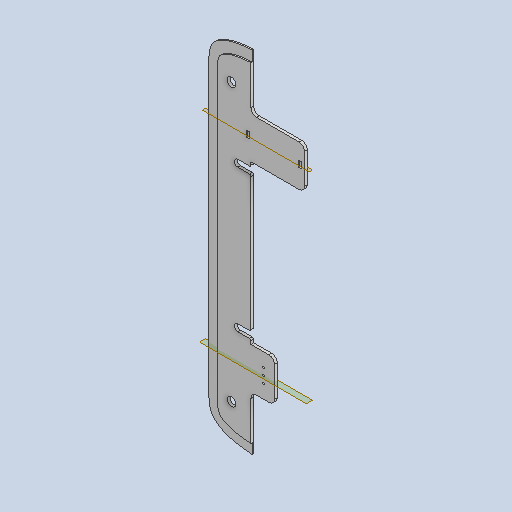
# Autodesk Inventor part: back_led_board
Saved by Autodesk Inventor 2022 (Build 260153000, 153)
## iProperties
Created: 2024-12-22
Part Number: back_led_board
Material: Типовые
Document SubType Name: Modeling
Designer: Andrey
Density: 1 g/cm^3
Appearance: По умолчанию
Author: Andrey
Autodesk Inventor part; units mm, degrees
ref_plane "YZ Plane" through (0, 0, 0) normal (1, 0, 0) x (0, 1, 0)
ref_plane "XZ Plane" through (0, 0, 0) normal (0, 1, 0) x (-1, 0, 0)
ref_plane "XY Plane" through (0, 0, 0) normal (0, 0, 1) x (1, 0, 0)
sketch "Эскиз1" plane through (0, 0, 0) normal (0, 0, 1) x (1, 0, 0)
  arc A0 (21.9698, 25.0872) -> (24.9698, 22.0872) centre (24.9698, 25.0872) ccw
  line L0 (24.9698, 22.0872) -> (32.4715, 22.0872)
  arc A1 (35.4715, 19.0872) -> (32.4715, 22.0872) centre (32.4715, 19.0872) ccw
  line L1 (35.4715, 19.0872) -> (35.4715, -12.1128)
  arc A2 (32.4715, -15.1128) -> (35.4715, -12.1128) centre (32.4715, -12.1128) ccw
  line L2 (32.4715, -15.1128) -> (24.9698, -15.1128)
  arc A3 (24.9698, -15.1128) -> (21.9698, -18.1128) centre (24.9698, -18.1128) ccw
  line L3 (21.9698, -18.1128) -> (21.9698, -28.1128)
  line L4 (21.9698, -28.1128) -> (36.9698, -28.1128)
  line L5 (36.9698, -28.1128) -> (36.9698, -40.6128)
  line L6 (36.9698, -40.6128) -> (21.9698, -40.6128)
  line L7 (21.9698, -40.6128) -> (21.9698, -43.5128)
  line L8 (21.9698, -43.5128) -> (58.0248, -43.5128)
  arc A4 (60.0248, -45.5128) -> (58.0248, -43.5128) centre (58.0248, -45.5128) ccw
  line L9 (60.0248, -45.5128) -> (60.0248, -60.8075)
  arc A5 (58.0248, -62.8075) -> (60.0248, -60.8075) centre (58.0248, -60.8075) ccw
  line L10 (58.0248, -62.8075) -> (-57.9752, -62.8075)
  arc A6 (-59.9752, -60.8075) -> (-57.9752, -62.8075) centre (-57.9752, -60.8075) ccw
  line L11 (-59.9752, -60.8075) -> (-59.9752, -45.5128)
  arc A7 (-57.9752, -43.5128) -> (-59.9752, -45.5128) centre (-57.9752, -45.5128) ccw
  line L12 (-57.9752, -43.5128) -> (-22.0457, -43.5128)
  line L13 (-22.0457, -43.5128) -> (-22.0457, -40.6128)
  line L14 (-22.0457, -40.6128) -> (-39.5957, -40.6128)
  line L15 (-39.5957, -40.6128) -> (-39.5957, -29.6128)
  line L16 (-39.5957, -29.6128) -> (-22.0457, -29.6128)
  line L17 (-22.0457, -29.6128) -> (-22.0457, -27.6266)
  line L18 (-22.0457, -27.6266) -> (-23.1715, -27.6266)
  line L19 (-23.1715, -27.6266) -> (-23.1715, -10.2508)
  line L20 (-23.1715, -10.2508) -> (-22.0457, -10.2508)
  line L21 (-22.0457, -10.2508) -> (-22.0457, -5.0128)
  line L22 (-22.0457, -5.0128) -> (-25.0457, -5.0128)
  line L23 (-25.0457, -5.0128) -> (-25.0457, 4.9872)
  line L24 (-25.0457, 4.9872) -> (-22.0457, 4.9872)
  line L25 (-22.0457, 4.9872) -> (-22.0457, 10.2252)
  line L26 (-22.0457, 10.2252) -> (-23.1715, 10.2252)
  line L27 (-23.1715, 10.2252) -> (-23.1715, 27.601)
  line L28 (-23.1715, 27.601) -> (-22.0457, 27.601)
  line L29 (-22.0457, 27.601) -> (-22.0457, 43.4872)
  line L30 (-22.0457, 43.4872) -> (-57.9752, 43.4872)
  arc A8 (-59.9752, 45.4872) -> (-57.9752, 43.4872) centre (-57.9752, 45.4872) ccw
  line L31 (-59.9752, 45.4872) -> (-59.9752, 60.782)
  arc A9 (-57.9752, 62.782) -> (-59.9752, 60.782) centre (-57.9752, 60.782) ccw
  line L32 (-57.9752, 62.782) -> (58.0248, 62.782)
  arc A10 (60.0248, 60.782) -> (58.0248, 62.782) centre (58.0248, 60.782) ccw
  line L33 (60.0248, 60.782) -> (60.0248, 45.4872)
  arc A11 (58.0248, 43.4872) -> (60.0248, 45.4872) centre (58.0248, 45.4872) ccw
  line L34 (58.0248, 43.4872) -> (21.9698, 43.4872)
  line L35 (21.9698, 43.4872) -> (21.9698, 25.0872)
  circle A12 centre (-51.6466, 22.9919) radius 1.5
  circle A13 centre (-51.6466, -23.0174) radius 1.5
  line L36 (-50.445, -3.8128) -> (-50.445, 15.6872)
  arc A14 (-47.445, 18.6872) -> (-50.445, 15.6872) centre (-47.445, 15.6872) ccw
  line L37 (-47.445, 18.6872) -> (-33.6813, 18.6872)
  arc A15 (-30.6813, 15.6872) -> (-33.6813, 18.6872) centre (-33.6813, 15.6872) ccw
  line L38 (-30.6813, 15.6872) -> (-30.6813, -3.8128)
  arc A16 (-33.6813, -6.8128) -> (-30.6813, -3.8128) centre (-33.6813, -3.8128) ccw
  line L39 (-33.6813, -6.8128) -> (-47.445, -6.8128)
  arc A17 (-50.445, -3.8128) -> (-47.445, -6.8128) centre (-47.445, -3.8128) ccw
  line L40 (60.4248, -29.3128) -> (60.4248, -21.9128)
  line L41 (60.4248, -21.9128) -> (74.9248, -21.9128)
  line L42 (74.9248, -21.9128) -> (74.9248, -29.3128)
  line L43 (74.9248, -29.3128) -> (60.4248, -29.3128)
  line L44 (60.4248, 21.8872) -> (60.4248, 29.2872)
  line L45 (60.4248, 29.2872) -> (74.9248, 29.2872)
  line L46 (74.9248, 29.2872) -> (74.9248, 21.8872)
  line L47 (74.9248, 21.8872) -> (60.4248, 21.8872)
  line L48 (79.0248, -17.5128) -> (68.0248, -17.5128)
  line L49 (68.0248, -17.5128) -> (68.0248, -6.0128)
  line L50 (68.0248, -6.0128) -> (63.1715, -6.0128)
  arc A18 (62.1715, -5.0128) -> (63.1715, -6.0128) centre (63.1715, -5.0128) ccw
  line L51 (62.1715, -5.0128) -> (62.1715, 4.9872)
  arc A19 (63.1715, 5.9872) -> (62.1715, 4.9872) centre (63.1715, 4.9872) ccw
  line L52 (63.1715, 5.9872) -> (68.0248, 5.9872)
  line L53 (68.0248, 5.9872) -> (68.0248, 17.4872)
  line L54 (68.0248, 17.4872) -> (79.0248, 17.4872)
  line L55 (79.0248, 17.4872) -> (79.0248, 52.7508)
  spline S0 degree 4 poles (79.0248, 52.7508) (79.0248, 55.4389) (78.6593, 58.1507) (77.2994, 60.4709) (75.0248, 62.2967) knots 0 0 0 0 0 1 1 1 1 1
  spline S1 degree 4 poles (75.0248, 62.2967) (71.8239, 64.8662) (66.8118, 66.4567) (60.2111, 66.782) (55.0248, 66.782) knots 0.415412 0.415412 0.415412 0.415412 0.415412 1 1 1 1 1
  line L56 (-54.9752, 66.782) -> (55.0248, 66.782)
  spline S2 degree 4 poles (-54.9752, 66.782) (-60.1615, 66.782) (-66.7622, 66.4567) (-71.7743, 64.8662) (-74.9752, 62.2967) knots 0 0 0 0 0 0.584588 0.584588 0.584588 0.584588 0.584588
  spline S3 degree 4 poles (-74.9752, 62.2967) (-77.2498, 60.4709) (-78.6098, 58.1507) (-78.9752, 55.4389) (-78.9752, 52.7508) knots 0 0 0 0 0 1 1 1 1 1
  line L57 (-78.9752, 52.7508) -> (-78.9752, -52.7764)
  spline S4 degree 4 poles (-78.9752, -52.7764) (-78.9752, -55.4644) (-78.6098, -58.1763) (-77.2498, -60.4964) (-74.9752, -62.3223) knots 0 0 0 0 0 1 1 1 1 1
  spline S5 degree 4 poles (-74.9752, -62.3223) (-71.7743, -64.8917) (-66.7622, -66.4822) (-60.1615, -66.8075) (-54.9752, -66.8075) knots 0.415412 0.415412 0.415412 0.415412 0.415412 1 1 1 1 1
  line L58 (55.0248, -66.8075) -> (-54.9752, -66.8075)
  spline S6 degree 4 poles (55.0248, -66.8075) (60.2111, -66.8075) (66.8118, -66.4822) (71.8239, -64.8917) (75.0248, -62.3223) knots 0 0 0 0 0 0.584588 0.584588 0.584588 0.584588 0.584588
  spline S7 degree 4 poles (75.0248, -62.3223) (77.2994, -60.4964) (78.6593, -58.1763) (79.0248, -55.4644) (79.0248, -52.7764) knots 0 0 0 0 0 1 1 1 1 1
  line L59 (79.0248, -52.7764) -> (79.0248, -17.5128)
  circle A20 centre (-29.4752, -25.5128) radius 1.25
  circle A21 centre (29.5248, 25.4872) radius 1.25
  circle A22 centre (29.5248, -25.5128) radius 1.25
  circle A23 centre (-29.4752, 25.4872) radius 1.25
  line L60 (-75.6752, -52.7764) -> (-75.6752, 52.7508)
  line L61 (-54.9752, 63.482) -> (55.0248, 63.482)
  line L62 (75.7248, 52.7508) -> (75.7248, 20.7872)
  line L63 (75.7248, 20.7872) -> (64.7248, 20.7872)
  line L64 (64.7248, 20.7872) -> (64.7248, 8.9969)
  arc A24 (64.7248, 8.9969) -> (58.8715, 4.9872) centre (63.1715, 4.9872) ccw
  line L65 (58.8715, 4.9872) -> (58.8715, -5.0128)
  arc A25 (58.8715, -5.0128) -> (64.7248, -9.0224) centre (63.1715, -5.0128) ccw
  line L66 (64.7248, -9.0224) -> (64.7248, -20.8128)
  line L67 (64.7248, -20.8128) -> (75.7248, -20.8128)
  line L68 (75.7248, -20.8128) -> (75.7248, -52.7764)
  line L69 (55.0248, -63.5075) -> (-54.9752, -63.5075)
  line L70 (-78.9752, 52.7508) -> (-78.9752, -52.7764)
  spline S8 degree 4 poles (-78.9752, -52.7764) (-78.9752, -55.4644) (-78.6098, -58.1763) (-77.2498, -60.4964) (-74.9752, -62.3223) knots 0 0 0 0 0 1 1 1 1 1
  spline S9 degree 4 poles (-74.9752, -62.3223) (-72.4991, -64.31) (-68.939, -65.7118) (-64.3981, -66.3953) (-59.9752, -66.667) knots 0 0 0 0 0 1 1 1 1 1
  line L71 (-59.9752, -66.667) -> (-59.9752, -28.4266)
  line L72 (-59.9752, -28.4266) -> (-75.9752, -28.4266)
  line L73 (-75.9752, -28.4266) -> (-75.9752, 28.401)
  line L74 (-75.9752, 28.401) -> (-59.9752, 28.401)
  line L75 (-59.9752, 28.401) -> (-59.9752, 66.6415)
  spline S10 degree 4 poles (-59.9752, 66.6415) (-64.3981, 66.3697) (-68.939, 65.6863) (-72.4991, 64.2844) (-74.9752, 62.2967) knots 0 0 0 0 0 1 1 1 1 1
  spline S11 degree 4 poles (-74.9752, 62.2967) (-77.2498, 60.4709) (-78.6098, 58.1507) (-78.9752, 55.4389) (-78.9752, 52.7508) knots 0 0 0 0 0 1 1 1 1 1
  line L76 (-78.9752, 52.7508) -> (-78.9752, -52.7764)
  spline S12 degree 4 poles (-74.9752, 62.2967) (-77.2498, 60.4709) (-78.6098, 58.1507) (-78.9752, 55.4389) (-78.9752, 52.7508) knots 0 0 0 0 0 1 1 1 1 1
  spline S13 degree 4 poles (-59.9752, 66.6415) (-64.3981, 66.3697) (-68.939, 65.6863) (-72.4991, 64.2844) (-74.9752, 62.2967) knots 0 0 0 0 0 1 1 1 1 1
  line L77 (-59.9752, 63.6356) -> (-59.9752, 66.6415)
  spline S14 degree 3 poles (-73.0972, 59.9572) (-72.8317, 60.1704) (-72.2504, 60.5866) (-71.3901, 61.0754) (-70.4297, 61.5347) (-69.5826, 61.8759) (-68.4322, 62.2648) (-67.4425, 62.5442) (-66.1307, 62.8516) (-65.027, 63.0635) (-63.595, 63.2862) (-62.4143, 63.4312) (-61.1039, 63.5554) (-60.3883, 63.6089) (-59.9752, 63.6356) knots 0 0 0 0 0.108911 0.217823 0.272278 0.38119 0.435645 0.544557 0.599012 0.707924 0.762379 0.871291 0.925747 1 1 1 1
  spline S15 degree 3 poles (-75.9752, 52.7508) (-75.9752, 53.2802) (-75.9431, 54.1752) (-75.8223, 55.1158) (-75.6926, 55.7827) (-75.5863, 56.208) (-75.4279, 56.7161) (-75.2804, 57.1045) (-75.0687, 57.5698) (-74.8765, 57.9272) (-74.6051, 58.3588) (-74.3614, 58.6932) (-74.0195, 59.1004) (-73.638, 59.4977) (-73.2859, 59.8058) (-73.0972, 59.9572) knots 0 0 0 0 0.166667 0.291667 0.333333 0.416667 0.458333 0.541667 0.583333 0.666667 0.708333 0.791667 0.833333 0.916667 1 1 1 1
  line L78 (-75.9752, -52.7764) -> (-75.9752, 52.7508)
  spline S16 degree 3 poles (-73.0972, -59.9828) (-73.2859, -59.8313) (-73.638, -59.5233) (-74.0195, -59.126) (-74.3614, -58.7188) (-74.6051, -58.3843) (-74.8765, -57.9527) (-75.0687, -57.5953) (-75.2804, -57.1301) (-75.4279, -56.7417) (-75.5863, -56.2336) (-75.6926, -55.8083) (-75.8007, -55.2525) (-75.8676, -54.7887) (-75.9281, -54.186) (-75.9662, -53.5615) (-75.9752, -53.0411) (-75.9752, -52.7764) knots 0 0 0 0 0.083333 0.166667 0.208333 0.291667 0.333333 0.416667 0.458333 0.541667 0.583333 0.666667 0.708333 0.791667 0.833333 0.916667 1 1 1 1
  spline S17 degree 3 poles (-59.9752, -63.6611) (-60.3883, -63.6345) (-61.1039, -63.581) (-62.4143, -63.4568) (-63.595, -63.3118) (-65.027, -63.0891) (-66.1307, -62.8772) (-67.4425, -62.5698) (-68.4322, -62.2903) (-69.5826, -61.9014) (-70.4297, -61.5602) (-71.3901, -61.101) (-72.2504, -60.6122) (-72.8317, -60.196) (-73.0972, -59.9828) knots 0 0 0 0 0.074253 0.128709 0.237621 0.292076 0.400988 0.455443 0.564355 0.61881 0.727722 0.782177 0.891089 1 1 1 1
  line L79 (-59.9752, -66.667) -> (-59.9752, -63.6611)
  spline S18 degree 4 poles (-74.9752, -62.3223) (-72.4991, -64.31) (-68.939, -65.7118) (-64.3981, -66.3953) (-59.9752, -66.667) knots 0 0 0 0 0 1 1 1 1 1
  spline S19 degree 4 poles (-78.9752, -52.7764) (-78.9752, -55.4644) (-78.6098, -58.1763) (-77.2498, -60.4964) (-74.9752, -62.3223) knots 0 0 0 0 0 1 1 1 1 1
  line L80 (-59.9752, -66.667) -> (-59.9752, 66.6415)
  spline S20 degree 5 poles (-54.9752, -63.5075) (-57.0934, -63.5074) (-59.2113, -63.4553) (-61.3274, -63.3195) (-65.0377, -62.9091) (-68.6545, -61.9829) (-70.1733, -61.4591) (-71.6562, -60.755) (-72.9094, -59.7489) knots 0 0 0 0 0 0 0.568819 0.568819 0.568819 1 1 1 1 1 1
  spline S21 degree 5 poles (-72.9094, -59.7489) (-73.483, -59.2877) (-74.0084, -58.7674) (-74.4613, -58.1707) (-75.2019, -56.783) (-75.5464, -55.2458) (-75.6371, -54.4235) (-75.6756, -53.6003) (-75.6752, -52.7764) knots 0 0 0 0 0 0 0.47184 0.47184 0.47184 1 1 1 1 1 1
  spline S22 degree 5 poles (-75.6752, 52.7508) (-75.6756, 53.5748) (-75.6371, 54.398) (-75.5464, 55.2203) (-75.2019, 56.7574) (-74.4613, 58.1451) (-74.0084, 58.7418) (-73.483, 59.2621) (-72.9094, 59.7233) knots 0 0 0 0 0 0 0.52816 0.52816 0.52816 1 1 1 1 1 1
  spline S23 degree 5 poles (-72.9094, 59.7233) (-71.6562, 60.7294) (-70.1733, 61.4336) (-68.6545, 61.9574) (-65.0377, 62.8835) (-61.3274, 63.2939) (-59.2113, 63.4297) (-57.0934, 63.4818) (-54.9752, 63.482) knots 0 0 0 0 0 0 0.431181 0.431181 0.431181 1 1 1 1 1 1
  spline S24 degree 5 poles (55.0248, 63.482) (57.143, 63.4818) (59.2609, 63.4297) (61.377, 63.2939) (65.0873, 62.8835) (68.704, 61.9574) (70.2229, 61.4336) (71.7058, 60.7294) (72.959, 59.7233) knots 0 0 0 0 0 0 0.568819 0.568819 0.568819 1 1 1 1 1 1
  spline S25 degree 5 poles (72.959, 59.7233) (73.5326, 59.2621) (74.0579, 58.7418) (74.5109, 58.1451) (75.2514, 56.7574) (75.596, 55.2203) (75.6867, 54.398) (75.7252, 53.5748) (75.7248, 52.7508) knots 0 0 0 0 0 0 0.47184 0.47184 0.47184 1 1 1 1 1 1
  spline S26 degree 5 poles (75.7248, -52.7764) (75.7252, -53.6003) (75.6867, -54.4235) (75.596, -55.2458) (75.2514, -56.783) (74.5109, -58.1707) (74.0579, -58.7674) (73.5326, -59.2877) (72.959, -59.7489) knots 0 0 0 0 0 0 0.52816 0.52816 0.52816 1 1 1 1 1 1
  spline S27 degree 5 poles (72.959, -59.7489) (71.7058, -60.755) (70.2229, -61.4591) (68.704, -61.9829) (65.0873, -62.9091) (61.377, -63.3195) (59.2609, -63.4553) (57.143, -63.5074) (55.0248, -63.5075) knots 0 0 0 0 0 0 0.431181 0.431181 0.431181 1 1 1 1 1 1
  point P0 (0, 0)
  point P1 (-59.9752, -63.3605)
  point P2 (-59.9752, 63.3349)
  dimension "d0" = 3.3
  constraints: 22 end point, 7 parallel, 4 point on circle, 2 centre point, 1 vertical, 32 other
extrude "Выдавливание1" add sketch "Эскиз1" along normal blind 1 contours L31 L75 L74 L60 S22 S23 | L80 L72 L60 L74 | L71 L11 S20 S21 L60 L72
sketch "Эскиз2" plane through (0, 0, 1) normal (0, 0, 1) x (1, 0, 0)
  line L0 (-44.445, -31.1128) -> (-44.445, -39.1128)
  arc A0 (-45.445, -40.1128) -> (-44.445, -39.1128) centre (-45.445, -39.1128) ccw
  line L1 (-45.445, -40.1128) -> (-48.445, -40.1128)
  arc A1 (-49.445, -39.1128) -> (-48.445, -40.1128) centre (-48.445, -39.1128) ccw
  line L2 (-49.445, -39.1128) -> (-49.445, -31.1128)
  arc A2 (-48.445, -30.1128) -> (-49.445, -31.1128) centre (-48.445, -31.1128) ccw
  line L3 (-48.445, -30.1128) -> (-45.445, -30.1128)
  arc A3 (-44.445, -31.1128) -> (-45.445, -30.1128) centre (-45.445, -31.1128) ccw
  circle A4 centre (-29.4752, 25.4872) radius 1.25
  circle A5 centre (29.5248, -25.5128) radius 1.25
  circle A6 centre (29.5248, 25.4872) radius 1.25
  circle A7 centre (-29.4752, -25.5128) radius 1.25
  line L4 (79.0248, -17.5128) -> (68.0248, -17.5128)
  line L5 (68.0248, -17.5128) -> (68.0248, -6.0128)
  line L6 (68.0248, -6.0128) -> (63.1715, -6.0128)
  arc A8 (62.1715, -5.0128) -> (63.1715, -6.0128) centre (63.1715, -5.0128) ccw
  line L7 (62.1715, -5.0128) -> (62.1715, 4.9872)
  arc A9 (63.1715, 5.9872) -> (62.1715, 4.9872) centre (63.1715, 4.9872) ccw
  line L8 (63.1715, 5.9872) -> (68.0248, 5.9872)
  line L9 (68.0248, 5.9872) -> (68.0248, 17.4872)
  line L10 (68.0248, 17.4872) -> (79.0248, 17.4872)
  line L11 (79.0248, 17.4872) -> (79.0248, 52.7508)
  spline S0 degree 4 poles (79.0248, 52.7508) (79.0248, 55.4389) (78.6593, 58.1507) (77.2994, 60.4709) (75.0248, 62.2967) knots 0 0 0 0 0 1 1 1 1 1
  spline S1 degree 4 poles (75.0248, 62.2967) (71.8239, 64.8662) (66.8118, 66.4567) (60.2111, 66.782) (55.0248, 66.782) knots 0.415412 0.415412 0.415412 0.415412 0.415412 1 1 1 1 1
  line L12 (-54.9752, 66.782) -> (55.0248, 66.782)
  spline S2 degree 4 poles (-54.9752, 66.782) (-60.1615, 66.782) (-66.7622, 66.4567) (-71.7743, 64.8662) (-74.9752, 62.2967) knots 0 0 0 0 0 0.584588 0.584588 0.584588 0.584588 0.584588
  spline S3 degree 4 poles (-74.9752, 62.2967) (-77.2498, 60.4709) (-78.6098, 58.1507) (-78.9752, 55.4389) (-78.9752, 52.7508) knots 0 0 0 0 0 1 1 1 1 1
  line L13 (-78.9752, 52.7508) -> (-78.9752, -52.7764)
  spline S4 degree 4 poles (-78.9752, -52.7764) (-78.9752, -55.4644) (-78.6098, -58.1763) (-77.2498, -60.4964) (-74.9752, -62.3223) knots 0 0 0 0 0 1 1 1 1 1
  spline S5 degree 4 poles (-74.9752, -62.3223) (-71.7743, -64.8917) (-66.7622, -66.4822) (-60.1615, -66.8075) (-54.9752, -66.8075) knots 0.415412 0.415412 0.415412 0.415412 0.415412 1 1 1 1 1
  line L14 (55.0248, -66.8075) -> (-54.9752, -66.8075)
  spline S6 degree 4 poles (55.0248, -66.8075) (60.2111, -66.8075) (66.8118, -66.4822) (71.8239, -64.8917) (75.0248, -62.3223) knots 0 0 0 0 0 0.584588 0.584588 0.584588 0.584588 0.584588
  spline S7 degree 4 poles (75.0248, -62.3223) (77.2994, -60.4964) (78.6593, -58.1763) (79.0248, -55.4644) (79.0248, -52.7764) knots 0 0 0 0 0 1 1 1 1 1
  line L15 (79.0248, -52.7764) -> (79.0248, -17.5128)
  line L16 (60.4248, 21.8872) -> (60.4248, 29.2872)
  line L17 (60.4248, 29.2872) -> (74.9248, 29.2872)
  line L18 (74.9248, 29.2872) -> (74.9248, 21.8872)
  line L19 (74.9248, 21.8872) -> (60.4248, 21.8872)
  line L20 (60.4248, -29.3128) -> (60.4248, -21.9128)
  line L21 (60.4248, -21.9128) -> (74.9248, -21.9128)
  line L22 (74.9248, -21.9128) -> (74.9248, -29.3128)
  line L23 (74.9248, -29.3128) -> (60.4248, -29.3128)
  circle A10 centre (-51.6466, -23.0174) radius 1.5
  circle A11 centre (-51.6466, 22.9919) radius 1.5
  arc A12 (21.9698, 25.0872) -> (24.9698, 22.0872) centre (24.9698, 25.0872) ccw
  line L24 (24.9698, 22.0872) -> (32.4715, 22.0872)
  arc A13 (35.4715, 19.0872) -> (32.4715, 22.0872) centre (32.4715, 19.0872) ccw
  line L25 (35.4715, 19.0872) -> (35.4715, -12.1128)
  arc A14 (32.4715, -15.1128) -> (35.4715, -12.1128) centre (32.4715, -12.1128) ccw
  line L26 (32.4715, -15.1128) -> (24.9698, -15.1128)
  arc A15 (24.9698, -15.1128) -> (21.9698, -18.1128) centre (24.9698, -18.1128) ccw
  line L27 (21.9698, -18.1128) -> (21.9698, -28.1128)
  line L28 (21.9698, -28.1128) -> (36.9698, -28.1128)
  line L29 (36.9698, -28.1128) -> (36.9698, -40.6128)
  line L30 (36.9698, -40.6128) -> (21.9698, -40.6128)
  line L31 (21.9698, -40.6128) -> (21.9698, -43.5128)
  line L32 (21.9698, -43.5128) -> (58.0248, -43.5128)
  arc A16 (60.0248, -45.5128) -> (58.0248, -43.5128) centre (58.0248, -45.5128) ccw
  line L33 (60.0248, -45.5128) -> (60.0248, -60.8075)
  arc A17 (58.0248, -62.8075) -> (60.0248, -60.8075) centre (58.0248, -60.8075) ccw
  line L34 (58.0248, -62.8075) -> (-57.9752, -62.8075)
  arc A18 (-59.9752, -60.8075) -> (-57.9752, -62.8075) centre (-57.9752, -60.8075) ccw
  line L35 (-59.9752, -60.8075) -> (-59.9752, -45.5128)
  arc A19 (-57.9752, -43.5128) -> (-59.9752, -45.5128) centre (-57.9752, -45.5128) ccw
  line L36 (-57.9752, -43.5128) -> (-22.0457, -43.5128)
  line L37 (-22.0457, -43.5128) -> (-22.0457, -40.6128)
  line L38 (-22.0457, -40.6128) -> (-39.5957, -40.6128)
  line L39 (-39.5957, -40.6128) -> (-39.5957, -29.6128)
  line L40 (-39.5957, -29.6128) -> (-22.0457, -29.6128)
  line L41 (-22.0457, -29.6128) -> (-22.0457, -27.6266)
  line L42 (-22.0457, -27.6266) -> (-23.1715, -27.6266)
  line L43 (-23.1715, -27.6266) -> (-23.1715, -10.2508)
  line L44 (-23.1715, -10.2508) -> (-22.0457, -10.2508)
  line L45 (-22.0457, -10.2508) -> (-22.0457, -5.0128)
  line L46 (-22.0457, -5.0128) -> (-25.0457, -5.0128)
  line L47 (-25.0457, -5.0128) -> (-25.0457, 4.9872)
  line L48 (-25.0457, 4.9872) -> (-22.0457, 4.9872)
  line L49 (-22.0457, 4.9872) -> (-22.0457, 10.2252)
  line L50 (-22.0457, 10.2252) -> (-23.1715, 10.2252)
  line L51 (-23.1715, 10.2252) -> (-23.1715, 27.601)
  line L52 (-23.1715, 27.601) -> (-22.0457, 27.601)
  line L53 (-22.0457, 27.601) -> (-22.0457, 43.4872)
  line L54 (-22.0457, 43.4872) -> (-57.9752, 43.4872)
  arc A20 (-59.9752, 45.4872) -> (-57.9752, 43.4872) centre (-57.9752, 45.4872) ccw
  line L55 (-59.9752, 45.4872) -> (-59.9752, 60.782)
  arc A21 (-57.9752, 62.782) -> (-59.9752, 60.782) centre (-57.9752, 60.782) ccw
  line L56 (-57.9752, 62.782) -> (58.0248, 62.782)
  arc A22 (60.0248, 60.782) -> (58.0248, 62.782) centre (58.0248, 60.782) ccw
  line L57 (60.0248, 60.782) -> (60.0248, 45.4872)
  arc A23 (58.0248, 43.4872) -> (60.0248, 45.4872) centre (58.0248, 45.4872) ccw
  line L58 (58.0248, 43.4872) -> (21.9698, 43.4872)
  line L59 (21.9698, 43.4872) -> (21.9698, 25.0872)
  arc A24 (-38.445, -6.8128) -> (-40.445, -8.8128) centre (-38.445, -8.8128) ccw
  line L60 (-40.445, -8.8128) -> (-40.445, -14.8128)
  arc A25 (-42.445, -16.8128) -> (-40.445, -14.8128) centre (-42.445, -14.8128) ccw
  line L61 (-42.445, -16.8128) -> (-48.445, -16.8128)
  arc A26 (-50.445, -14.8128) -> (-48.445, -16.8128) centre (-48.445, -14.8128) ccw
  line L62 (-50.445, -14.8128) -> (-50.445, 15.6872)
  arc A27 (-47.445, 18.6872) -> (-50.445, 15.6872) centre (-47.445, 15.6872) ccw
  line L63 (-47.445, 18.6872) -> (-33.6813, 18.6872)
  arc A28 (-30.6813, 15.6872) -> (-33.6813, 18.6872) centre (-33.6813, 15.6872) ccw
  line L64 (-30.6813, 15.6872) -> (-30.6813, -3.8128)
  arc A29 (-33.6813, -6.8128) -> (-30.6813, -3.8128) centre (-33.6813, -3.8128) ccw
  line L65 (-33.6813, -6.8128) -> (-38.445, -6.8128)
  line L66 (-78.9752, -28.1266) -> (-39.8957, -28.1266)
  line L67 (-39.8957, 28.101) -> (-78.9752, 28.101)
  line L68 (-75.6752, 52.7508) -> (-75.6752, -52.7764)
  line L69 (-59.9752, -63.3605) -> (-59.9752, 63.3349)
  line L70 (-78.9752, -28.6266) -> (-39.5957, -28.6266)
  line L71 (-39.5957, 28.601) -> (-78.9752, 28.601)
  line L72 (-39.5957, 20.7141) -> (-39.5957, 66.782)
  line L73 (-39.5957, 43.4872) -> (-39.5957, -43.5128)
  line L74 (-51.445, -28.6266) -> (-51.445, -43.5128)
  line L75 (-40.5957, 43.4872) -> (-40.5957, -43.5128)
  line L76 (-59.9752, -63.3605) -> (-59.9752, 63.3349)
  line L77 (-59.9752, -28.6266) -> (-51.445, -28.6266)
  line L78 (-55.445, -28.6266) -> (-55.445, -43.5128)
  circle A30 centre (-55.445, -32.5697) radius 1.5
  circle A31 centre (-55.445, -39.5697) radius 1.5
  line L79 (-55.445, -39.5697) -> (-55.445, -32.5697)
  line L80 (-56.945, -32.5697) -> (-56.945, -39.5697)
  line L81 (-53.945, -39.5697) -> (-53.945, -32.5697)
  line L82 (-56.945, -39.5697) -> (-56.945, -32.5697)
  arc A32 (-53.945, -32.5697) -> (-56.945, -32.5697) centre (-55.445, -32.5697) ccw
  line L83 (-53.945, -32.5697) -> (-53.945, -39.5697)
  arc A33 (-56.945, -39.5697) -> (-53.945, -39.5697) centre (-55.445, -39.5697) ccw
  point P0 (0, 0)
  point P1 (-55.445, -36.0697)
  point P2 (-40.5957, 28.601)
  point P3 (-59.9752, 45.4872)
  point P4 (-59.9752, 28.601)
  point P5 (-59.9752, -28.6266)
  dimension "d3" = 0.5
  dimension "d4" = 0.5
  dimension "d5" = 2
  dimension "d6" = 1
  dimension "d7" = 3
  dimension "d8" = 3
  dimension "d9" = 7
  dimension "d10" = 4
  constraints: 20 end point, 13 point on line, 4 point on circle, 4 tangent, 3 parallel, 3 perpendicular, 2 centre point, 2 collinear, 2 midpoint, 4 other
  measures "d3" distance between parallel lines of L66 L70
  measures "d4" distance between parallel lines of L67 L71
  measures "d5" distance between parallel lines of L2 L74
  measures "d6" distance between parallel lines of L73 L75
  measures "d7" diameter of A30
  measures "d8" diameter of A31
  measures "d9" distance of L79.start L79.end
  measures "d10" distance between parallel lines of L74 L78
extrude "Выдавливание2" add sketch "Эскиз2" against normal blind 1 contours L70 L78 A30 L80 A31 L36 A19 L69 | L70 L74 L36 L78 A31 L81 A30 | A30 L78 | L78 A30 | L69 A20 L54 L75 L71 | L81 A31 L78 A30 | A30 L78 A31 L80 | A31 L78 | L78 A31
fillet "Сопряжение1" radius 2 4 edges at (-40.5957, 43.4872, 0.5) (-40.5957, 28.601, 0.5) (-51.445, -43.5128, 0.5) (-51.445, -28.6266, 0.5)
ref_plane "РабПлоскость1" through (-57.9752, -36.0697, 1) normal (0, -1, 0) x (1, 0, 0)
sketch "Эскиз3" plane through (0, 0, 1) normal (0, 0, 1) x (1, 0, 0)
  line L0 (-59.9752, -28.6266) -> (-59.9752, 28.601) projected
  line L1 (-75.6752, 52.7508) -> (-75.6752, -52.7764) projected
  arc A0 (-51.445, -30.6266) -> (-53.445, -28.6266) centre (-53.445, -30.6266) ccw projected
  line L2 (-53.445, -28.6266) -> (-59.9752, -28.6266) projected
  line L3 (-59.9752, -28.6266) -> (-59.9752, 28.601) projected
  line L4 (-59.9752, 28.601) -> (-42.5957, 28.601) projected
  arc A1 (-42.5957, 28.601) -> (-40.5957, 30.601) centre (-42.5957, 30.601) ccw projected
  line L5 (-40.5957, 30.601) -> (-40.5957, 41.4872) projected
  arc A2 (-40.5957, 41.4872) -> (-42.5957, 43.4872) centre (-42.5957, 41.4872) ccw projected
  line L6 (-42.5957, 43.4872) -> (-57.9752, 43.4872) projected
  arc A3 (-59.9752, 45.4872) -> (-57.9752, 43.4872) centre (-57.9752, 45.4872) ccw projected
  line L7 (-59.9752, 45.4872) -> (-59.9752, 63.3349) projected
  line L8 (-75.6752, 52.7508) -> (-75.6752, -52.7764) projected
  line L9 (-59.9752, -63.3605) -> (-59.9752, -45.5128) projected
  arc A4 (-57.9752, -43.5128) -> (-59.9752, -45.5128) centre (-57.9752, -45.5128) ccw projected
  line L10 (-57.9752, -43.5128) -> (-53.445, -43.5128) projected
  arc A5 (-53.445, -43.5128) -> (-51.445, -41.5128) centre (-53.445, -41.5128) ccw projected
  line L11 (-51.445, -41.5128) -> (-51.445, -30.6266) projected
  line L12 (-66.9752, -62.3689) -> (-66.9752, 62.3433)
  line L13 (-66.9752, -0.0128) -> (-66.9752, -50.0128)
  circle A6 centre (-66.9752, -50.0128) radius 1.6
  line L14 (-66.9752, -0.0128) -> (-66.9752, 49.9872)
  circle A7 centre (-66.9752, 49.9872) radius 1.6
  line L15 (-59.9752, -0.0128) -> (-75.6752, -0.0128)
  point P0 (0, 0)
  dimension "d14" = 50
  dimension "d15" = 3.2
  dimension "d16" = 50
  dimension "d17" = 3.2
  dimension "d18" = 7
  constraints: 8 end point, 3 midpoint, 3 point on line, 2 centre point, 2 coincident, 1 vertical, 6 other
  measures "d14" distance of L13.start L13.end
  measures "d15" diameter of A6
  measures "d16" distance of L13.start L14.end
  measures "d17" diameter of A7
  measures "d18" distance between parallel lines of L12 L0
extrude "Выдавливание3" cut sketch "Эскиз3" against normal blind 1
sketch "Эскиз4" plane through (0, 0, 0) normal (0, 0, -1) x (-1, 0, 0)
  line L0 (60.8752, -26.0128) -> (60.8752, 25.9872)
  line L1 (73.8752, 25.9872) -> (73.8752, -26.0128)
  line L2 (70.8752, -29.0128) -> (63.8752, -29.0128)
  arc A0 (60.8752, -26.0128) -> (63.8752, -29.0128) centre (63.8752, -26.0128) ccw
  circle A1 centre (66.9752, -50.0128) radius 1.35
  circle A2 centre (66.9752, 49.9872) radius 1.35
  arc A3 (57.945, -33.5297) -> (52.945, -33.5297) centre (55.445, -33.5297) ccw
  line L3 (57.945, -33.5297) -> (57.945, -38.6097)
  arc A4 (52.945, -38.6097) -> (57.945, -38.6097) centre (55.445, -38.6097) ccw
  line L4 (52.945, -38.6097) -> (52.945, -33.5297)
  line L5 (44.445, -39.1128) -> (44.445, -31.1128)
  arc A5 (45.445, -30.1128) -> (44.445, -31.1128) centre (45.445, -31.1128) ccw
  line L6 (45.445, -30.1128) -> (48.445, -30.1128)
  arc A6 (49.445, -31.1128) -> (48.445, -30.1128) centre (48.445, -31.1128) ccw
  line L7 (49.445, -31.1128) -> (49.445, -39.1128)
  arc A7 (48.445, -40.1128) -> (49.445, -39.1128) centre (48.445, -39.1128) ccw
  line L8 (48.445, -40.1128) -> (45.445, -40.1128)
  arc A8 (44.445, -39.1128) -> (45.445, -40.1128) centre (45.445, -39.1128) ccw
  arc A9 (40.445, -8.8128) -> (38.445, -6.8128) centre (38.445, -8.8128) ccw
  line L9 (38.445, -6.8128) -> (33.6813, -6.8128)
  arc A10 (30.6813, -3.8128) -> (33.6813, -6.8128) centre (33.6813, -3.8128) ccw
  line L10 (30.6813, -3.8128) -> (30.6813, 15.6872)
  arc A11 (33.6813, 18.6872) -> (30.6813, 15.6872) centre (33.6813, 15.6872) ccw
  line L11 (33.6813, 18.6872) -> (47.445, 18.6872)
  arc A12 (50.445, 15.6872) -> (47.445, 18.6872) centre (47.445, 15.6872) ccw
  line L12 (50.445, 15.6872) -> (50.445, -14.8128)
  arc A13 (48.445, -16.8128) -> (50.445, -14.8128) centre (48.445, -14.8128) ccw
  line L13 (48.445, -16.8128) -> (42.445, -16.8128)
  arc A14 (40.445, -14.8128) -> (42.445, -16.8128) centre (42.445, -14.8128) ccw
  line L14 (40.445, -14.8128) -> (40.445, -8.8128)
  circle A15 centre (51.6466, 22.9919) radius 1.5
  circle A16 centre (51.6466, -23.0174) radius 1.5
  line L15 (-60.4248, -21.9128) -> (-60.4248, -29.3128)
  line L16 (-60.4248, -29.3128) -> (-74.9248, -29.3128)
  line L17 (-74.9248, -29.3128) -> (-74.9248, -21.9128)
  line L18 (-74.9248, -21.9128) -> (-60.4248, -21.9128)
  line L19 (-60.4248, 29.2872) -> (-60.4248, 21.8872)
  line L20 (-60.4248, 21.8872) -> (-74.9248, 21.8872)
  line L21 (-74.9248, 21.8872) -> (-74.9248, 29.2872)
  line L22 (-74.9248, 29.2872) -> (-60.4248, 29.2872)
  line L23 (-68.0248, -17.5128) -> (-79.0248, -17.5128)
  line L24 (-79.0248, -52.7764) -> (-79.0248, -17.5128)
  spline S0 degree 4 poles (-75.0248, -62.3223) (-77.2994, -60.4964) (-78.6593, -58.1763) (-79.0248, -55.4644) (-79.0248, -52.7764) knots 0 0 0 0 0 1 1 1 1 1
  spline S1 degree 4 poles (-55.0248, -66.8075) (-60.2111, -66.8075) (-66.8118, -66.4822) (-71.8239, -64.8917) (-75.0248, -62.3223) knots 0 0 0 0 0 0.584588 0.584588 0.584588 0.584588 0.584588
  line L25 (54.9752, -66.8075) -> (-55.0248, -66.8075)
  spline S2 degree 4 poles (74.9752, -62.3223) (71.7743, -64.8917) (66.7622, -66.4822) (60.1615, -66.8075) (54.9752, -66.8075) knots 0.415412 0.415412 0.415412 0.415412 0.415412 1 1 1 1 1
  spline S3 degree 4 poles (78.9752, -52.7764) (78.9752, -55.4644) (78.6098, -58.1763) (77.2498, -60.4964) (74.9752, -62.3223) knots 0 0 0 0 0 1 1 1 1 1
  line L26 (78.9752, 52.7508) -> (78.9752, -52.7764)
  spline S4 degree 4 poles (74.9752, 62.2967) (77.2498, 60.4709) (78.6098, 58.1507) (78.9752, 55.4389) (78.9752, 52.7508) knots 0 0 0 0 0 1 1 1 1 1
  spline S5 degree 4 poles (54.9752, 66.782) (60.1615, 66.782) (66.7622, 66.4567) (71.7743, 64.8662) (74.9752, 62.2967) knots 0 0 0 0 0 0.584588 0.584588 0.584588 0.584588 0.584588
  line L27 (-55.0248, 66.782) -> (54.9752, 66.782)
  spline S6 degree 4 poles (-75.0248, 62.2967) (-71.8239, 64.8662) (-66.8118, 66.4567) (-60.2111, 66.782) (-55.0248, 66.782) knots 0.415412 0.415412 0.415412 0.415412 0.415412 1 1 1 1 1
  spline S7 degree 4 poles (-79.0248, 52.7508) (-79.0248, 55.4389) (-78.6593, 58.1507) (-77.2994, 60.4709) (-75.0248, 62.2967) knots 0 0 0 0 0 1 1 1 1 1
  line L28 (-79.0248, 17.4872) -> (-79.0248, 52.7508)
  line L29 (-79.0248, 17.4872) -> (-68.0248, 17.4872)
  line L30 (-68.0248, 17.4872) -> (-68.0248, 5.9872)
  line L31 (-68.0248, 5.9872) -> (-63.1715, 5.9872)
  arc A17 (-62.1715, 4.9872) -> (-63.1715, 5.9872) centre (-63.1715, 4.9872) ccw
  line L32 (-62.1715, 4.9872) -> (-62.1715, -5.0128)
  arc A18 (-63.1715, -6.0128) -> (-62.1715, -5.0128) centre (-63.1715, -5.0128) ccw
  line L33 (-63.1715, -6.0128) -> (-68.0248, -6.0128)
  line L34 (-68.0248, -6.0128) -> (-68.0248, -17.5128)
  circle A19 centre (29.4752, -25.5128) radius 1.25
  circle A20 centre (-29.5248, 25.4872) radius 1.25
  circle A21 centre (-29.5248, -25.5128) radius 1.25
  circle A22 centre (29.4752, 25.4872) radius 1.25
  arc A23 (-24.9698, 22.0872) -> (-21.9698, 25.0872) centre (-24.9698, 25.0872) ccw
  line L35 (-21.9698, 25.0872) -> (-21.9698, 43.4872)
  line L36 (-58.0248, 43.4872) -> (-21.9698, 43.4872)
  arc A24 (-60.0248, 45.4872) -> (-58.0248, 43.4872) centre (-58.0248, 45.4872) ccw
  line L37 (-60.0248, 45.4872) -> (-60.0248, 60.782)
  arc A25 (-58.0248, 62.782) -> (-60.0248, 60.782) centre (-58.0248, 60.782) ccw
  line L38 (-58.0248, 62.782) -> (57.9752, 62.782)
  arc A26 (59.9752, 60.782) -> (57.9752, 62.782) centre (57.9752, 60.782) ccw
  line L39 (59.9752, 60.782) -> (59.9752, 45.4872)
  arc A27 (57.9752, 43.4872) -> (59.9752, 45.4872) centre (57.9752, 45.4872) ccw
  line L40 (22.0457, 43.4872) -> (57.9752, 43.4872)
  line L41 (22.0457, 43.4872) -> (22.0457, 27.601)
  line L42 (22.0457, 27.601) -> (23.1715, 27.601)
  line L43 (23.1715, 27.601) -> (23.1715, 10.2252)
  line L44 (23.1715, 10.2252) -> (22.0457, 10.2252)
  line L45 (22.0457, 10.2252) -> (22.0457, 4.9872)
  line L46 (22.0457, 4.9872) -> (25.0457, 4.9872)
  line L47 (25.0457, 4.9872) -> (25.0457, -5.0128)
  line L48 (25.0457, -5.0128) -> (22.0457, -5.0128)
  line L49 (22.0457, -5.0128) -> (22.0457, -10.2508)
  line L50 (22.0457, -10.2508) -> (23.1715, -10.2508)
  line L51 (23.1715, -10.2508) -> (23.1715, -27.6266)
  line L52 (23.1715, -27.6266) -> (22.0457, -27.6266)
  line L53 (22.0457, -27.6266) -> (22.0457, -29.6128)
  line L54 (22.0457, -29.6128) -> (39.5957, -29.6128)
  line L55 (39.5957, -29.6128) -> (39.5957, -40.6128)
  line L56 (39.5957, -40.6128) -> (22.0457, -40.6128)
  line L57 (22.0457, -40.6128) -> (22.0457, -43.5128)
  line L58 (57.9752, -43.5128) -> (22.0457, -43.5128)
  arc A28 (59.9752, -45.5128) -> (57.9752, -43.5128) centre (57.9752, -45.5128) ccw
  line L59 (59.9752, -45.5128) -> (59.9752, -60.8075)
  arc A29 (57.9752, -62.8075) -> (59.9752, -60.8075) centre (57.9752, -60.8075) ccw
  line L60 (57.9752, -62.8075) -> (-58.0248, -62.8075)
  arc A30 (-60.0248, -60.8075) -> (-58.0248, -62.8075) centre (-58.0248, -60.8075) ccw
  line L61 (-60.0248, -60.8075) -> (-60.0248, -45.5128)
  arc A31 (-58.0248, -43.5128) -> (-60.0248, -45.5128) centre (-58.0248, -45.5128) ccw
  line L62 (-21.9698, -43.5128) -> (-58.0248, -43.5128)
  line L63 (-21.9698, -43.5128) -> (-21.9698, -40.6128)
  line L64 (-21.9698, -40.6128) -> (-36.9698, -40.6128)
  line L65 (-36.9698, -40.6128) -> (-36.9698, -28.1128)
  line L66 (-36.9698, -28.1128) -> (-21.9698, -28.1128)
  line L67 (-21.9698, -28.1128) -> (-21.9698, -18.1128)
  arc A32 (-21.9698, -18.1128) -> (-24.9698, -15.1128) centre (-24.9698, -18.1128) ccw
  line L68 (-24.9698, -15.1128) -> (-32.4715, -15.1128)
  arc A33 (-35.4715, -12.1128) -> (-32.4715, -15.1128) centre (-32.4715, -12.1128) ccw
  line L69 (-35.4715, -12.1128) -> (-35.4715, 19.0872)
  arc A34 (-32.4715, 22.0872) -> (-35.4715, 19.0872) centre (-32.4715, 19.0872) ccw
  line L70 (-32.4715, 22.0872) -> (-24.9698, 22.0872)
  circle A35 centre (66.9752, 49.9872) radius 1.6
  circle A36 centre (66.9752, -50.0128) radius 1.6
  arc A37 (53.445, -28.6266) -> (51.445, -30.6266) centre (53.445, -30.6266) ccw
  line L71 (53.445, -28.6266) -> (59.9752, -28.6266)
  line L72 (59.9752, -28.6266) -> (59.9752, 28.601)
  line L73 (59.9752, 28.601) -> (42.5957, 28.601)
  arc A38 (40.5957, 30.601) -> (42.5957, 28.601) centre (42.5957, 30.601) ccw
  line L74 (40.5957, 30.601) -> (40.5957, 41.4872)
  arc A39 (42.5957, 43.4872) -> (40.5957, 41.4872) centre (42.5957, 41.4872) ccw
  line L75 (42.5957, 43.4872) -> (57.9752, 43.4872)
  arc A40 (57.9752, 43.4872) -> (59.9752, 45.4872) centre (57.9752, 45.4872) ccw
  line L76 (59.9752, 45.4872) -> (59.9752, 63.3349)
  line L77 (75.6752, 52.7508) -> (75.6752, -52.7764)
  line L78 (59.9752, -63.3605) -> (59.9752, -45.5128)
  arc A41 (59.9752, -45.5128) -> (57.9752, -43.5128) centre (57.9752, -45.5128) ccw
  line L79 (57.9752, -43.5128) -> (53.445, -43.5128)
  arc A42 (51.445, -41.5128) -> (53.445, -43.5128) centre (53.445, -41.5128) ccw
  line L80 (51.445, -41.5128) -> (51.445, -30.6266)
  line L81 (73.9752, -28.1266) -> (59.6752, -28.1266)
  ellipse E0 centre (45.8066, 13.1872) end of major axis (31.7723, 13.1872) minor radius 4.8 (59.8409, 13.1872) -> (59.6752, 13.9225) ccw
  line L82 (59.8409, -1.3128) -> (59.8409, 13.1872)
  ellipse E1 centre (45.8066, -1.3128) end of major axis (59.8409, -1.3128) minor radius 4.8 (59.6752, -2.0481) -> (59.8409, -1.3128) ccw
  line L83 (59.6752, -28.1266) -> (59.6752, -2.0481)
  line L84 (73.9752, -28.1266) -> (59.6752, -28.1266)
  line L85 (73.9752, 28.101) -> (73.9752, -28.1266)
  line L86 (59.6752, 28.101) -> (73.9752, 28.101)
  line L87 (59.6752, 13.9225) -> (59.6752, 28.101)
  arc A43 (63.8752, 28.9872) -> (60.8752, 25.9872) centre (63.8752, 25.9872) ccw
  line L88 (63.8752, 28.9872) -> (70.8752, 28.9872)
  arc A44 (73.8752, 25.9872) -> (70.8752, 28.9872) centre (70.8752, 25.9872) ccw
  arc A45 (70.8752, -29.0128) -> (73.8752, -26.0128) centre (70.8752, -26.0128) ccw
  circle A46 centre (70.8752, 25.9872) radius 1
  circle A47 centre (70.8752, -26.0128) radius 1
  line L89 (55.9752, 24.4872) -> (55.9752, 28.101)
  line L90 (39.8957, 28.101) -> (55.9752, 28.101)
  line L91 (39.8957, 28.101) -> (39.8957, 16.9648)
  ellipse E2 centre (48.5541, 13.1872) end of major axis (34.5198, 13.1872) minor radius 4.8 (59.6752, 16.115) -> (39.8957, 16.9648) ccw
  line L92 (59.6752, 16.115) -> (59.6752, 24.4872)
  line L93 (59.6752, 24.4872) -> (55.9752, 24.4872)
  circle A48 centre (51.6466, 22.9919) radius 2.1
  line L94 (59.9752, 26.9872) -> (71.3752, 26.9872)
  line L95 (71.3752, 24.4872) -> (59.6752, 24.4872)
  line L96 (71.3752, -27.0128) -> (60.2174, -27.0128)
  line L97 (59.6752, -24.5128) -> (71.3752, -24.5128)
  line L98 (59.9752, -28.6266) -> (59.9752, 28.601)
  line L99 (59.9752, -24.5128) -> (65.9752, -24.5128)
  line L100 (65.9752, -24.5128) -> (65.9752, -27.0128)
  line L101 (65.9752, -27.0128) -> (59.9752, -27.0128)
  line L102 (59.9752, -27.0128) -> (59.9752, -24.5128)
  line L103 (59.9752, 24.4872) -> (65.9752, 24.4872)
  line L104 (65.9752, 24.4872) -> (65.9752, 26.9872)
  line L105 (65.9752, 26.9872) -> (59.9752, 26.9872)
  line L106 (59.9752, 26.9872) -> (59.9752, 24.4872)
  point P0 (0, 0)
  dimension "d21" = 2
  dimension "d22" = 2
  dimension "d25" = 6
  constraints: 16 end point, 6 point on line, 4 parallel, 2 centre point, 2 coincident, 2 horizontal, 2 perpendicular, 1 collinear, 7 other
  measures "d21" diameter of A46
  measures "d22" diameter of A47
  measures "d25" distance between parallel lines of L72 L104
extrude "Выдавливание4" cut sketch "Эскиз4" against normal blind 10 contours A0 L96 L101 L72 L97 L0 | L0 L97 L100 L96 A0 | L95 L72 L94 A43 L0 | L0 A43 L94 L104 L95
ref_plane "РабПлоскость2" through (-57.9752, 36.0441, 1) normal (0, 1, 0) x (1, 0, 0)
fillet "Сопряжение2" radius 1.25 4 edges at (-65.9752, -24.5128, 0.5) (-65.9752, -27.0128, 0.5) (-65.9752, 26.9872, 0.5) (-65.9752, 24.4872, 0.5)
fillet "Сопряжение3" radius 0.5 4 edges at (-59.9752, 26.9872, 0.5) (-59.9752, 24.4872, 0.5) (-59.9752, -27.0128, 0.5) (-59.9752, -24.5128, 0.5)
sketch "Эскиз5" plane through (0, 0, 1) normal (0, 0, 1) x (1, 0, 0)
  line L0 (-55.665, -38.8297) -> (-55.225, -38.8297)
  line L1 (-55.225, -38.8297) -> (-55.225, -38.3897)
  line L2 (-55.225, -38.3897) -> (-55.665, -38.3897)
  line L3 (-55.665, -38.3897) -> (-55.665, -38.8297)
  line L4 (-55.665, -36.2897) -> (-55.225, -36.2897)
  line L5 (-55.225, -36.2897) -> (-55.225, -35.8497)
  line L6 (-55.225, -35.8497) -> (-55.665, -35.8497)
  line L7 (-55.665, -35.8497) -> (-55.665, -36.2897)
  line L8 (-55.665, -33.7497) -> (-55.225, -33.7497)
  line L9 (-55.225, -33.7497) -> (-55.225, -33.3097)
  line L10 (-55.225, -33.3097) -> (-55.665, -33.3097)
  line L11 (-55.665, -33.3097) -> (-55.665, -33.7497)
  line L12 (-71.9752, 52.7508) -> (-71.9752, 28.401)
  line L13 (-71.9752, 28.401) -> (-75.9752, 28.401)
  line L14 (-75.9752, 52.7508) -> (-75.9752, 28.401)
  spline S0 degree 3 poles (-73.0972, 59.9572) (-73.6185, 59.5388) (-74.0864, 59.066) (-74.8459, 58.0248) (-75.1323, 57.4882) (-75.8259, 55.6628) (-75.9752, 54.268) (-75.9752, 52.7508) knots -0.895425 -0.895425 -0.895425 -0.895425 -0.666738 -0.666738 -0.455136 -0.455136 0 0 0 0
  spline S1 degree 3 poles (-59.9752, 63.6356) (-63.0917, 63.4346) (-66.5976, 62.9677) (-70.7785, 61.423) (-72.0475, 60.7999) (-73.0972, 59.9572) knots -1.341069 -1.341069 -1.341069 -1.341069 -0.403833 -0.403833 0 0 0 0
  line L15 (-59.9752, 63.6356) -> (-59.9752, 59.6267)
  spline S2 degree 3 poles (-59.9752, 59.6267) (-60.3216, 59.6027) (-61.0961, 59.5418) (-62.0646, 59.4425) (-63.0897, 59.3145) (-63.8834, 59.196) (-64.8353, 59.028) (-65.5612, 58.8782) (-66.4153, 58.6735) (-67.0551, 58.4965) (-67.7186, 58.2859) (-68.1284, 58.1402) (-68.512, 57.9912) (-68.7543, 57.8906) (-69.0394, 57.7643) (-69.2537, 57.6628) (-69.5043, 57.5363) (-69.6911, 57.4354) (-69.9079, 57.3106) (-70.0677, 57.2122) (-70.2511, 57.0918) (-70.419, 56.9738) (-70.5377, 56.8826) (-70.5933, 56.8379) knots 0 0 0 0 0.067932 0.152665 0.195032 0.279766 0.322132 0.406866 0.449233 0.533966 0.576333 0.639883 0.661066 0.703433 0.724616 0.766983 0.788166 0.830533 0.851716 0.894083 0.915267 0.957633 1 1 1 1
  spline S3 degree 3 poles (-70.5933, 56.8379) (-70.6449, 56.7965) (-70.7419, 56.7151) (-70.8489, 56.6174) (-70.9464, 56.5224) (-71.0171, 56.4489) (-71.0978, 56.359) (-71.1568, 56.2887) (-71.2383, 56.1847) (-71.3108, 56.0826) (-71.3987, 55.9429) (-71.4584, 55.8351) (-71.5153, 55.7201) (-71.5519, 55.6399) (-71.5962, 55.5337) (-71.6305, 55.4436) (-71.672, 55.3231) (-71.7041, 55.2203) (-71.7427, 55.0829) (-71.7721, 54.9653) (-71.8069, 54.8083) (-71.833, 54.6746) (-71.863, 54.4969) (-71.8849, 54.3458) (-71.9093, 54.1461) (-71.9262, 53.9782) (-71.9474, 53.7134) (-71.9686, 53.3347) (-71.9752, 52.9693) (-71.9752, 52.7508) knots 0 0 0 0 0.041667 0.083333 0.104167 0.145833 0.166667 0.208333 0.229167 0.291667 0.333333 0.395833 0.416667 0.458333 0.479167 0.520833 0.541667 0.583333 0.604167 0.645833 0.666667 0.708333 0.729167 0.770833 0.791667 0.833333 0.854167 0.916667 1 1 1 1
  spline S4 degree 3 poles (-70.5933, -56.8635) (-70.5377, -56.9081) (-70.419, -56.9993) (-70.2511, -57.1174) (-70.0677, -57.2378) (-69.9079, -57.3362) (-69.6911, -57.461) (-69.5043, -57.5619) (-69.2537, -57.6884) (-69.0394, -57.7899) (-68.7543, -57.9162) (-68.512, -58.0167) (-68.1284, -58.1657) (-67.7186, -58.3115) (-67.0551, -58.5221) (-66.4153, -58.6991) (-65.5612, -58.9037) (-64.8353, -59.0536) (-63.8834, -59.2216) (-63.0897, -59.3401) (-62.0646, -59.4681) (-61.0961, -59.5674) (-60.3216, -59.6283) (-59.9752, -59.6522) knots 0 0 0 0 0.042367 0.084733 0.105917 0.148284 0.169467 0.211834 0.233017 0.275384 0.296567 0.338934 0.360117 0.423667 0.466034 0.550767 0.593134 0.677868 0.720234 0.804968 0.847335 0.932068 1 1 1 1
  line L16 (-59.9752, -59.6522) -> (-59.9752, -63.6611)
  spline S5 degree 3 poles (-73.0972, -59.9828) (-72.4152, -60.5303) (-71.6452, -60.9817) (-69.882, -61.8156) (-68.8367, -62.1777) (-65.3082, -63.1528) (-62.5505, -63.4951) (-59.9752, -63.6611) knots -1.360047 -1.360047 -1.360047 -1.360047 -1.097743 -1.097743 -0.7742 -0.7742 0 0 0 0
  spline S6 degree 3 poles (-75.9752, -52.7764) (-75.9752, -53.6959) (-75.9207, -54.6418) (-75.5876, -56.3375) (-75.34, -57.0946) (-74.5444, -58.5559) (-73.9595, -59.2906) (-73.0972, -59.9828) knots -1.001631 -1.001631 -1.001631 -1.001631 -0.643463 -0.643463 -0.331719 -0.331719 0 0 0 0
  line L17 (-75.9752, -28.4266) -> (-75.9752, -52.7764)
  line L18 (-75.9752, -28.4266) -> (-71.9752, -28.4266)
  line L19 (-71.9752, -28.4266) -> (-71.9752, -52.7764)
  spline S7 degree 3 poles (-71.9752, -52.7764) (-71.9752, -52.886) (-71.9733, -53.1001) (-71.9662, -53.3537) (-71.9533, -53.6449) (-71.9346, -53.9198) (-71.8966, -54.2979) (-71.8525, -54.6002) (-71.7939, -54.9007) (-71.7504, -55.081) (-71.7041, -55.2459) (-71.672, -55.3487) (-71.6305, -55.4692) (-71.5962, -55.5592) (-71.5519, -55.6654) (-71.5153, -55.7457) (-71.4584, -55.8607) (-71.3987, -55.9684) (-71.3108, -56.1082) (-71.2383, -56.2103) (-71.1568, -56.3143) (-71.0978, -56.3846) (-71.0171, -56.4745) (-70.9464, -56.548) (-70.8489, -56.6429) (-70.7419, -56.7407) (-70.6449, -56.822) (-70.5933, -56.8635) knots 0 0 0 0 0.041667 0.083333 0.104167 0.166667 0.208333 0.291667 0.333333 0.395833 0.416667 0.458333 0.479167 0.520833 0.541667 0.583333 0.604167 0.666667 0.708333 0.770833 0.791667 0.833333 0.854167 0.895833 0.916667 0.958333 1 1 1 1
  line L20 (-71.9752, -28.4266) -> (-71.9752, 28.401)
  line L21 (-75.9752, 28.401) -> (-75.9752, -28.4266)
  line L22 (-75.6752, 52.7508) -> (-75.6752, -52.7764)
  line L23 (-42.7757, 37.6441) -> (-42.7757, 35.4441)
  line L24 (-42.7757, 35.4441) -> (-41.7957, 35.4441)
  line L25 (-41.7957, 35.4441) -> (-41.5957, 35.6441)
  line L26 (-41.5957, 37.4441) -> (-41.5957, 35.6441)
  line L27 (-41.7957, 37.6441) -> (-41.5957, 37.4441)
  line L28 (-42.7757, 37.6441) -> (-41.7957, 37.6441)
  line L29 (-61.5457, 37.6441) -> (-61.7457, 37.4441)
  line L30 (-61.7457, 37.4441) -> (-61.7457, 35.6441)
  line L31 (-61.5457, 35.4441) -> (-61.7457, 35.6441)
  line L32 (-61.5457, 35.4441) -> (-60.5657, 35.4441)
  line L33 (-60.5657, 37.6441) -> (-60.5657, 35.4441)
  line L34 (-61.5457, 37.6441) -> (-60.5657, 37.6441)
  line L35 (-55.665, -38.8297) -> (-55.225, -38.3897)
  line L36 (-55.665, -36.2897) -> (-55.225, -35.8497)
  line L37 (-55.665, -33.7497) -> (-55.225, -33.3097)
  circle A0 centre (-55.445, -38.6097) radius 0.375
  circle A1 centre (-55.445, -36.0697) radius 0.375
  circle A2 centre (-55.445, -33.5297) radius 0.375
  point P0 (0, 0)
extrude "Выдавливание5" cut sketch "Эскиз5" against normal blind 0.5 contours L35 L1 L0 | L3 L2 L35 | L36 L5 L4 | L7 L6 L36 | L37 L9 L8 | L11 L10 L37 | L12 L13 L14 S0 S1 L15 S2 S3 | L20 L18 L22 L13 | L22 L18 L21 L13 | L19 S7 S4 L16 S5 S6 L17 L18 | L28 L27 L26 L25 L24 L23 | L34 L33 L32 L31 L30 L29 | A0 | A1 | A2
